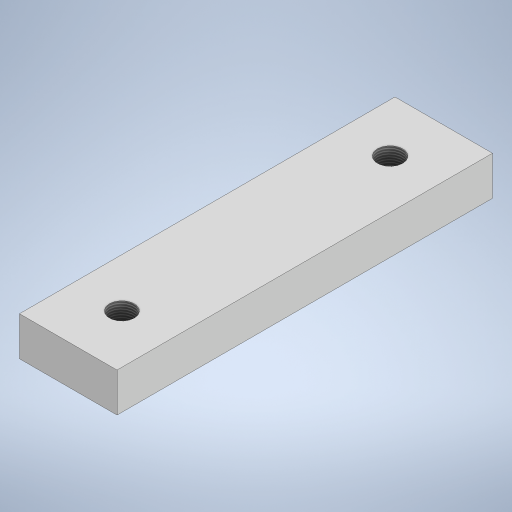
# Autodesk Inventor part: Spannbacke(n)
Saved by Autodesk Inventor 2024 (Build 280153000, 153)
## iProperties
Created: 2023-05-10
Part Number: Spannbacke(n)
Material: Generic
Document SubType Name: Modeling
Designer: dell
Density: 1 g/cm^3
Appearance: Default
Author: dell
Autodesk Inventor part; units mm, degrees
ref_plane "YZ Plane" through (0, 0, 0) normal (1, 0, 0) x (0, 1, 0)
ref_plane "XZ Plane" through (0, 0, 0) normal (0, 1, 0) x (-1, 0, 0)
ref_plane "XY Plane" through (0, 0, 0) normal (0, 0, 1) x (1, 0, 0)
sketch "Sketch1" plane through (0, 0, 0) normal (0, 1, 0) x (-1, 0, 0)
  line L0 (10, 38.5) -> (-10, 38.5)
  line L1 (-10, 38.5) -> (-10, -38.5)
  line L2 (-10, -38.5) -> (10, -38.5)
  line L3 (10, -38.5) -> (10, 38.5)
  line L4 (10, 38.5) -> (-10, -38.5) construction
  line L5 (-10, 38.5) -> (10, -38.5) construction
  point P0 (0, 0)
  dimension "d0" = 77
  dimension "d1" = 20
  constraints: 12 end point, 2 midpoint, 2 parallel, 1 horizontal, 1 perpendicular
  measures "d0" distance of L2.end L0.start
  measures "d1" distance of L0.start L0.end
extrude "Extrusion1" add sketch "Sketch1" along normal blind 8
sketch "Sketch3" plane through (0, 8, 0) normal (0, 1, 0) x (1, 0, 0)
  circle A0 centre (0, -27.5) radius 2.5574
  circle A1 centre (0, 27.5) radius 2.6
  point P0 (0, 0)
  dimension "d8" = 5.2
  dimension "d9" = 55
  dimension "d10" = 27.5
  constraints: 2 centre point
  measures "d8" diameter of A1
  measures "d9" distance of A0.centre A1.centre
  measures "d10" distance of point (0, 0) A0.centre
extrude "Extrusion2" cut sketch "Sketch3" against normal blind 6
thread "Thread1" size "M5.5x0.5" class "6H" standard "ANSI Metric M Profile" full length
thread "Thread2" size "M5.5x0.5" class "6H" standard "ANSI Metric M Profile" full length
body "Solid1"
